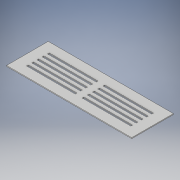
# Autodesk Inventor part: 16 inch grill
Saved by Autodesk Inventor 2017 (Build 210142000, 142)
## iProperties
Created: 2017-08-29
Part Number: 16 inch grill
Material: Generic
Document SubType Name: Modeling
Designer: mcgratta
Density: 1 g/cm^3
Appearance: Default
Author: mcgratta
Autodesk Inventor part; units mm, degrees
ref_plane "YZ Plane" through (0, 0, 0) normal (1, 0, 0) x (0, 1, 0)
ref_plane "XZ Plane" through (0, 0, 0) normal (0, 1, 0) x (-1, 0, 0)
ref_plane "XY Plane" through (0, 0, 0) normal (0, 0, 1) x (1, 0, 0)
sketch "Sketch1" plane through (0, 0, 0) normal (0, 1, 0) x (-1, 0, 0)
  line L0 (0, 0) -> (-457.2, 0)
  line L1 (-457.2, 0) -> (-457.2, -152.4)
  line L2 (-457.2, -152.4) -> (0, -152.4)
  line L3 (0, -152.4) -> (0, 0)
  line L4 (-25.4, -25.4) -> (-431.8, -25.4)
  line L5 (-431.8, -25.4) -> (-431.8, -127)
  line L6 (-431.8, -127) -> (-25.4, -127)
  line L7 (-25.4, -127) -> (-25.4, -25.4)
  line L8 (-38.1, -117.475) -> (-215.9, -117.475)
  line L9 (-215.9, -117.475) -> (-215.9, -111.125)
  line L10 (-215.9, -111.125) -> (-38.1, -111.125)
  line L11 (-38.1, -111.125) -> (-38.1, -117.475)
  line L12 (-38.1, -98.425) -> (-215.9, -98.425)
  line L13 (-215.9, -98.425) -> (-215.9, -92.075)
  line L14 (-215.9, -92.075) -> (-38.1, -92.075)
  line L15 (-38.1, -92.075) -> (-38.1, -98.425)
  line L16 (-38.1, -79.375) -> (-215.9, -79.375)
  line L17 (-215.9, -79.375) -> (-215.9, -73.025)
  line L18 (-215.9, -73.025) -> (-38.1, -73.025)
  line L19 (-38.1, -73.025) -> (-38.1, -79.375)
  line L20 (-38.1, -60.325) -> (-215.9, -60.325)
  line L21 (-215.9, -60.325) -> (-215.9, -53.975)
  line L22 (-215.9, -53.975) -> (-38.1, -53.975)
  line L23 (-38.1, -53.975) -> (-38.1, -60.325)
  line L24 (-38.1, -41.275) -> (-215.9, -41.275)
  line L25 (-215.9, -41.275) -> (-215.9, -34.925)
  line L26 (-215.9, -34.925) -> (-38.1, -34.925)
  line L27 (-38.1, -34.925) -> (-38.1, -41.275)
  line L28 (-241.3, -117.475) -> (-419.1, -117.475)
  line L29 (-419.1, -117.475) -> (-419.1, -111.125)
  line L30 (-419.1, -111.125) -> (-241.3, -111.125)
  line L31 (-241.3, -111.125) -> (-241.3, -117.475)
  line L32 (-241.3, -92.075) -> (-241.3, -98.425)
  line L33 (-241.3, -98.425) -> (-419.1, -98.425)
  line L34 (-419.1, -98.425) -> (-419.1, -92.075)
  line L35 (-419.1, -92.075) -> (-241.3, -92.075)
  line L36 (-241.3, -73.025) -> (-241.3, -79.375)
  line L37 (-241.3, -79.375) -> (-419.1, -79.375)
  line L38 (-419.1, -79.375) -> (-419.1, -73.025)
  line L39 (-419.1, -73.025) -> (-241.3, -73.025)
  line L40 (-241.3, -53.975) -> (-241.3, -60.325)
  line L41 (-241.3, -60.325) -> (-419.1, -60.325)
  line L42 (-419.1, -60.325) -> (-419.1, -53.975)
  line L43 (-419.1, -53.975) -> (-241.3, -53.975)
  line L44 (-241.3, -34.925) -> (-241.3, -41.275)
  line L45 (-241.3, -41.275) -> (-419.1, -41.275)
  line L46 (-419.1, -41.275) -> (-419.1, -34.925)
  line L47 (-419.1, -34.925) -> (-241.3, -34.925)
  dimension "d0" = 457.2
  dimension "d1" = 152.4
  dimension "d2" = 25.4
  dimension "d3" = 25.4
  dimension "d4" = 25.4
  dimension "d5" = 25.4
  dimension "d6" = 6.35
  dimension "d7" = 12.7
  dimension "d8" = 9.525
  dimension "d9" = 177.8
  dimension "d10" = 6.35
  dimension "d11" = 177.8
  dimension "d12" = 6.35
  dimension "d13" = 177.8
  dimension "d14" = 6.35
  dimension "d15" = 177.8
  dimension "d16" = 6.35
  dimension "d17" = 177.8
  dimension "d18" = 12.7
  dimension "d19" = 12.7
  dimension "d20" = 12.7
  dimension "d21" = 12.7
  dimension "d22" = 12.7
  dimension "d23" = 12.7
  dimension "d24" = 12.7
  dimension "d25" = 12.7
  dimension "d26" = 6.35
  dimension "d27" = 177.8
  dimension "d28" = 6.35
  dimension "d29" = 177.8
  dimension "d30" = 6.35
  dimension "d31" = 177.8
  dimension "d32" = 6.35
  dimension "d33" = 177.8
  dimension "d34" = 6.35
  dimension "d35" = 177.8
  dimension "d36" = 12.7
  dimension "d37" = 12.7
  dimension "d38" = 12.7
  dimension "d39" = 12.7
  dimension "d68" = 9.525
  dimension "d69" = 25.4
  dimension "d70" = 25.4
  dimension "d71" = 25.4
  dimension "d72" = 25.4
  dimension "d73" = 25.4
  constraints: 96 end point, 24 parallel, 12 horizontal, 12 perpendicular
  measures "d0" distance of L1.end L2.end
  measures "d1" distance of L0.end L1.end
  measures "d2" distance between parallel lines of L3 L7
  measures "d3" distance between parallel lines of L6 L2
  measures "d4" distance between parallel lines of L0 L4
  measures "d5" distance between parallel lines of L1 L5
  measures "d6" distance between parallel lines of L10 L8
  measures "d7" distance between parallel lines of L11 L7
  measures "d8" distance between parallel lines of L8 L6
  measures "d9" distance between parallel lines of L9 L11
  measures "d10" distance between parallel lines of L14 L12
  measures "d11" distance between parallel lines of L13 L15
  measures "d12" distance between parallel lines of L18 L16
  measures "d13" distance between parallel lines of L17 L19
  measures "d14" distance between parallel lines of L22 L20
  measures "d15" distance between parallel lines of L21 L23
  measures "d16" distance between parallel lines of L26 L24
  measures "d17" distance between parallel lines of L25 L27
  measures "d18" distance between parallel lines of L12 L10
  measures "d19" distance between parallel lines of L16 L14
  measures "d20" distance between parallel lines of L20 L18
  measures "d21" distance between parallel lines of L24 L22
  measures "d22" distance between parallel lines of L15 L7
  measures "d23" distance between parallel lines of L19 L7
  measures "d24" distance between parallel lines of L7 L23
  measures "d25" distance between parallel lines of L7 L27
  measures "d26" distance between parallel lines of L30 L28
  measures "d27" distance between parallel lines of L29 L31
  measures "d28" distance between parallel lines of L35 L33
  measures "d29" distance between parallel lines of L34 L32
  measures "d30" distance between parallel lines of L39 L37
  measures "d31" distance between parallel lines of L38 L36
  measures "d32" distance between parallel lines of L43 L41
  measures "d33" distance between parallel lines of L42 L40
  measures "d34" distance between parallel lines of L47 L45
  measures "d35" distance between parallel lines of L46 L44
  measures "d36" distance between parallel lines of L33 L30
  measures "d37" distance between parallel lines of L37 L35
  measures "d38" distance between parallel lines of L41 L39
  measures "d39" distance between parallel lines of L45 L43
  measures "d68" distance between parallel lines of L28 L6
  measures "d69" distance between parallel lines of L31 L9
  measures "d70" distance between parallel lines of L32 L13
  measures "d71" distance between parallel lines of L36 L17
  measures "d72" distance between parallel lines of L40 L21
  measures "d73" distance between parallel lines of L44 L25
extrude "Extrusion2" add sketch "Sketch1" along normal blind 3.175 contours L3 L2 L1 L0 | L7 L6 L5 L4
body "Solid2"
